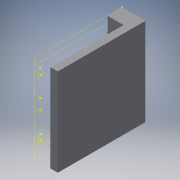
# Autodesk Inventor part: AXTS
Saved by Autodesk Inventor 2016 (Build 200138000, 138)
## iProperties
Created: 2017-07-16
Part Number: AXTS
Material: PC/ABS Plastic
Document SubType Name: Modeling
Designer: ludwi
Density: 0.357273 g/cm^3
Appearance: Smooth - White
Author: ludwi
Autodesk Inventor part; units mm, degrees
ref_plane "YZ Plane" through (0, 0, 0) normal (1, 0, 0) x (0, 1, 0)
ref_plane "XZ Plane" through (0, 0, 0) normal (0, 1, 0) x (-1, 0, 0)
ref_plane "XY Plane" through (0, 0, 0) normal (0, 0, 1) x (1, 0, 0)
sketch "Sketch1" plane through (0, 0, 0) normal (0, 0, 1) x (1, 0, 0)
  line L0 (0, 0) -> (32, 0)
  line L1 (32, 0) -> (32, -120)
  line L2 (32, -120) -> (22, -120)
  line L3 (22, -120) -> (22, -20)
  line L4 (22, -20) -> (0, -20)
  line L5 (0, -20) -> (0, 0)
  dimension "d3" = 120
  dimension "d4" = 10
  dimension "d5" = 22
  dimension "d8" = 20
  constraints: 12 end point, 4 perpendicular, 1 horizontal, 1 vertical
  measures "d3" distance of L0.end L1.end
  measures "d4" distance of L1.end L2.end
  measures "d5" horizontal distance of L0.start L2.end
  measures "d8" distance of L4.end L0.start
extrude "Extrusion1" add sketch "Sketch1" against normal blind 120
sketch "Sketch3" plane through (0, -20, 0) normal (-1, 0, 0) x (0, 0, 1)
  line L0 (-110, -97.8692) -> (-110, 18.1308) construction
  line L1 (-10, 18.1308) -> (-10, -97.8692) construction
  line L2 (-25, 8.9558) -> (-17, 8.9558) construction
  arc A0 (-17, 8.9558) -> (-17, 15.0558) centre (-17, 12.0058) ccw construction
  line L3 (-17, 15.0558) -> (-25, 15.0558) construction
  arc A1 (-25, 15.0558) -> (-25, 8.9558) centre (-25, 12.0058) ccw construction
  line L4 (-25, -94.7942) -> (-17, -94.7942) construction
  arc A2 (-17, -94.7942) -> (-17, -88.6942) centre (-17, -91.7442) ccw construction
  line L5 (-17, -88.6942) -> (-25, -88.6942) construction
  arc A3 (-25, -88.6942) -> (-25, -94.7942) centre (-25, -91.7442) ccw construction
  circle A4 centre (-25, -50.2442) radius 3.05 construction
  circle A5 centre (-25, -29.4942) radius 3.05 construction
  circle A6 centre (-95, -29.4942) radius 3.05 construction
  circle A7 centre (-95, -50.2442) radius 3.05 construction
  line L6 (-95, 15.0558) -> (-103, 15.0558) construction
  arc A8 (-103, 15.0558) -> (-103, 8.9558) centre (-103, 12.0058) ccw construction
  line L7 (-103, 8.9558) -> (-95, 8.9558) construction
  arc A9 (-95, 8.9558) -> (-95, 15.0558) centre (-95, 12.0058) ccw construction
  circle A10 centre (-67.125, 12.0058) radius 3.05 construction
  line L8 (-52.875, -32.5442) -> (-44.875, -32.5442) construction
  arc A11 (-44.875, -32.5442) -> (-44.875, -26.4442) centre (-44.875, -29.4942) ccw construction
  line L9 (-44.875, -26.4442) -> (-52.875, -26.4442) construction
  arc A12 (-52.875, -26.4442) -> (-52.875, -32.5442) centre (-52.875, -29.4942) ccw construction
  circle A13 centre (-52.875, -91.7442) radius 3.05 construction
  circle A14 centre (-52.875, 12.0058) radius 3.05 construction
  line L10 (-52.875, -53.2942) -> (-44.875, -53.2942) construction
  arc A15 (-44.875, -53.2942) -> (-44.875, -47.1942) centre (-44.875, -50.2442) ccw construction
  line L11 (-44.875, -47.1942) -> (-52.875, -47.1942) construction
  arc A16 (-52.875, -47.1942) -> (-52.875, -53.2942) centre (-52.875, -50.2442) ccw construction
  circle A17 centre (-67.125, -91.7442) radius 3.05 construction
  line L12 (-75.125, -53.2942) -> (-67.125, -53.2942) construction
  arc A18 (-67.125, -53.2942) -> (-67.125, -47.1942) centre (-67.125, -50.2442) ccw construction
  line L13 (-67.125, -47.1942) -> (-75.125, -47.1942) construction
  arc A19 (-75.125, -47.1942) -> (-75.125, -53.2942) centre (-75.125, -50.2442) ccw construction
  line L14 (-103, -94.7942) -> (-95, -94.7942) construction
  arc A20 (-95, -94.7942) -> (-95, -88.6942) centre (-95, -91.7442) ccw construction
  line L15 (-95, -88.6942) -> (-103, -88.6942) construction
  arc A21 (-103, -88.6942) -> (-103, -94.7942) centre (-103, -91.7442) ccw construction
  line L16 (-75.125, -32.5442) -> (-67.125, -32.5442) construction
  arc A22 (-67.125, -32.5442) -> (-67.125, -26.4442) centre (-67.125, -29.4942) ccw construction
  line L17 (-67.125, -26.4442) -> (-75.125, -26.4442) construction
  arc A23 (-75.125, -26.4442) -> (-75.125, -32.5442) centre (-75.125, -29.4942) ccw construction
  line L18 (0, -100) -> (0, 0) construction
  line L19 (0, 0) -> (-120, 0) construction
  line L20 (-120, -100) -> (-120, 0) construction
  line L21 (0, -100) -> (-120, -100) construction
  line L22 (0, 0) -> (0, 20) construction
  line L23 (0, 20) -> (-120, 20) construction
  line L24 (-120, 0) -> (-120, 20) construction
  line L25 (0, 0) -> (-120, 0) construction
  line L26 (-120, 0) -> (-110, -10)
  line L27 (-110, -99.8692) -> (-110, -10)
  line L28 (0, -100) -> (-120, -100) projected
  line L29 (-120, -100) -> (-110, -99.8692)
  line L30 (-120, -100) -> (-120, 0)
  line L31 (-120, 20) -> (-120, -100) projected
  line L32 (0, 0) -> (-120, 0) projected
  line L33 (0, 0) -> (-10, -10)
  line L34 (-10, -10) -> (-10, -99.8692)
  line L35 (0, 20) -> (0, -100) projected
  line L36 (-10, -99.8692) -> (0, -100)
  line L37 (0, -100) -> (0, -100)
  line L38 (0, 0) -> (0, -100)
  line L39 (-120, -98.4303) -> (-110, -98.4303)
  line L40 (-110, -98.4303) -> (-110, -107.1574)
  line L41 (-110, -107.1574) -> (-120, -107.1574)
  line L42 (-120, -107.1574) -> (-120, -98.4303)
  line L43 (0, -94.7942) -> (-10, -94.7942)
  line L44 (-10, -94.7942) -> (-10, -110)
  line L45 (-10, -110) -> (0, -110)
  line L46 (0, -110) -> (0, -94.7942)
  line L47 (-10, 18.1308) -> (-110, 18.1308) projected
  line L48 (-110, -97.8692) -> (-10, -97.8692) projected
  point P0 (-213, 15.0558)
  point P1 (-213, -88.6942)
  point P2 (-127, 8.9558)
  point P3 (-185.125, -26.4442)
  point P4 (-185.125, -47.1942)
  point P5 (-162.875, -47.1942)
  point P6 (-135, -88.6942)
  point P7 (-162.875, -26.4442)
  dimension "d12" = 135
  dimension "d13" = 135
  constraints: 34 end point, 4 parallel, 4 point on line, 3 perpendicular, 2 collinear, 2 horizontal
  measures "d12" angle of L35 L33
  measures "d13" angle of L20 L26
extrude "Extrusion2" cut sketch "Sketch3" against normal through all contours L26 L27 L39 L30 | L39 L27 L29 L30 | L35 L43 L34 L33 | L29 L40 L28 | L28 L40 L41 L42 | L35 L36 L34 L43 | L46 L45 L44 L28 | L28 L44 L36
chamfer "Chamfer2" distance 2 angle 45 6 edges at (22, -20, -60) (0, -20, -60) (0, 0, -60) (32, 0, -60) (32, -120, -60) (22, -120, -60)
sketch "Sketch4" plane through (2, -20, -120) normal (0, -1, 0) x (1, 0, 0)
  line L0 (98.1462, 2) -> (-1.8538, 2) construction
  line L1 (98.1462, 2) -> (98.1462, 118) construction
  line L2 (-1.8538, 118) -> (98.1462, 118) construction
  line L3 (-1.8538, 118) -> (-1.8538, 2) construction
  line L4 (83.1462, 11.175) -> (91.1462, 11.175) construction
  arc A0 (91.1462, 5.075) -> (91.1462, 11.175) centre (91.1462, 8.125) ccw construction
  line L5 (91.1462, 5.075) -> (83.1462, 5.075) construction
  arc A1 (83.1462, 11.175) -> (83.1462, 5.075) centre (83.1462, 8.125) ccw construction
  line L6 (83.1462, 114.925) -> (91.1462, 114.925) construction
  arc A2 (91.1462, 108.825) -> (91.1462, 114.925) centre (91.1462, 111.875) ccw construction
  line L7 (91.1462, 108.825) -> (83.1462, 108.825) construction
  arc A3 (83.1462, 114.925) -> (83.1462, 108.825) centre (83.1462, 111.875) ccw construction
  circle A4 centre (83.1462, 70.375) radius 3.05 construction
  circle A5 centre (83.1462, 49.625) radius 3.05 construction
  circle A6 centre (13.1462, 49.625) radius 3.05 construction
  circle A7 centre (13.1462, 70.375) radius 3.05 construction
  line L8 (13.1462, 5.075) -> (5.1462, 5.075) construction
  arc A8 (5.1462, 11.175) -> (5.1462, 5.075) centre (5.1462, 8.125) ccw construction
  line L9 (5.1462, 11.175) -> (13.1462, 11.175) construction
  arc A9 (13.1462, 5.075) -> (13.1462, 11.175) centre (13.1462, 8.125) ccw construction
  circle A10 centre (41.0212, 8.125) radius 3.05 construction
  line L10 (55.2712, 52.675) -> (63.2712, 52.675) construction
  arc A11 (63.2712, 46.575) -> (63.2712, 52.675) centre (63.2712, 49.625) ccw construction
  line L11 (63.2712, 46.575) -> (55.2712, 46.575) construction
  arc A12 (55.2712, 52.675) -> (55.2712, 46.575) centre (55.2712, 49.625) ccw construction
  circle A13 centre (55.2712, 111.875) radius 3.05 construction
  circle A14 centre (55.2712, 8.125) radius 3.05 construction
  line L12 (55.2712, 73.425) -> (63.2712, 73.425) construction
  arc A15 (63.2712, 67.325) -> (63.2712, 73.425) centre (63.2712, 70.375) ccw construction
  line L13 (63.2712, 67.325) -> (55.2712, 67.325) construction
  arc A16 (55.2712, 73.425) -> (55.2712, 67.325) centre (55.2712, 70.375) ccw construction
  circle A17 centre (41.0212, 111.875) radius 3.05 construction
  line L14 (33.0212, 73.425) -> (41.0212, 73.425) construction
  arc A18 (41.0212, 67.325) -> (41.0212, 73.425) centre (41.0212, 70.375) ccw construction
  line L15 (41.0212, 67.325) -> (33.0212, 67.325) construction
  arc A19 (33.0212, 73.425) -> (33.0212, 67.325) centre (33.0212, 70.375) ccw construction
  line L16 (5.1462, 114.925) -> (13.1462, 114.925) construction
  arc A20 (13.1462, 108.825) -> (13.1462, 114.925) centre (13.1462, 111.875) ccw construction
  line L17 (13.1462, 108.825) -> (5.1462, 108.825) construction
  arc A21 (5.1462, 114.925) -> (5.1462, 108.825) centre (5.1462, 111.875) ccw construction
  line L18 (33.0212, 52.675) -> (41.0212, 52.675) construction
  arc A22 (41.0212, 46.575) -> (41.0212, 52.675) centre (41.0212, 49.625) ccw construction
  line L19 (41.0212, 46.575) -> (33.0212, 46.575) construction
  arc A23 (33.0212, 52.675) -> (33.0212, 46.575) centre (33.0212, 49.625) ccw construction
  line L20 (13.1462, 49.625) -> (5.1462, 49.625) construction
  line L21 (13.1462, 46.575) -> (5.1462, 46.575)
  line L22 (5.1462, 52.675) -> (13.1462, 52.675)
  arc A24 (13.1462, 46.575) -> (13.1462, 52.675) centre (13.1462, 49.625) ccw
  arc A25 (5.1462, 52.675) -> (5.1462, 46.575) centre (5.1462, 49.625) ccw
  line L23 (13.1462, 70.375) -> (5.1462, 70.375) construction
  line L24 (13.1462, 67.325) -> (5.1462, 67.325)
  line L25 (5.1462, 73.425) -> (13.1462, 73.425)
  arc A26 (13.1462, 67.325) -> (13.1462, 73.425) centre (13.1462, 70.375) ccw
  arc A27 (5.1462, 73.425) -> (5.1462, 67.325) centre (5.1462, 70.375) ccw
  line L26 (13.1462, 111.875) -> (5.1462, 111.875) construction
  line L27 (13.1462, 108.825) -> (5.1462, 108.825)
  line L28 (5.1462, 114.925) -> (13.1462, 114.925)
  arc A28 (13.1462, 108.825) -> (13.1462, 114.925) centre (13.1462, 111.875) ccw
  arc A29 (5.1462, 114.925) -> (5.1462, 108.825) centre (5.1462, 111.875) ccw
  line L29 (13.1462, 8.125) -> (5.1462, 8.125) construction
  line L30 (13.1462, 5.075) -> (5.1462, 5.075)
  line L31 (5.1462, 11.175) -> (13.1462, 11.175)
  arc A30 (13.1462, 5.075) -> (13.1462, 11.175) centre (13.1462, 8.125) ccw
  arc A31 (5.1462, 11.175) -> (5.1462, 5.075) centre (5.1462, 8.125) ccw
  point P0 (-2, 120)
  point P1 (9.1462, 49.625)
  point P2 (9.1462, 70.375)
  point P3 (9.1462, 111.875)
  point P4 (9.1462, 8.125)
  constraints: 32 end point, 16 point on circle, 16 tangent, 8 centre point, 7 parallel, 4 midpoint, 2 concentric, 1 horizontal
sketch "Sketch5" plane through (22, -118, -10) normal (-1, 0, 0) x (0, 0, 1)
  line L0 (0, 116.1308) -> (-100, 116.1308) projected
  line L1 (0, 116.1308) -> (0, 0.1308) projected
  line L2 (-100, 0.1308) -> (0, 0.1308) projected
  line L3 (-100, 0.1308) -> (-100, 116.1308) projected
  line L4 (-15, 106.9558) -> (-7, 106.9558) projected
  arc A0 (-7, 106.9558) -> (-7, 113.0558) centre (-7, 110.0058) ccw projected
  line L5 (-7, 113.0558) -> (-15, 113.0558) projected
  arc A1 (-15, 113.0558) -> (-15, 106.9558) centre (-15, 110.0058) ccw projected
  line L6 (-15, 3.2058) -> (-7, 3.2058) projected
  arc A2 (-7, 3.2058) -> (-7, 9.3058) centre (-7, 6.2558) ccw projected
  line L7 (-7, 9.3058) -> (-15, 9.3058) projected
  arc A3 (-15, 9.3058) -> (-15, 3.2058) centre (-15, 6.2558) ccw projected
  circle A4 centre (-15, 47.7558) radius 3.05 projected
  circle A5 centre (-15, 68.5058) radius 3.05 projected
  circle A6 centre (-85, 68.5058) radius 3.05 projected
  circle A7 centre (-85, 47.7558) radius 3.05 projected
  line L8 (-85, 113.0558) -> (-93, 113.0558) projected
  arc A8 (-93, 113.0558) -> (-93, 106.9558) centre (-93, 110.0058) ccw projected
  line L9 (-93, 106.9558) -> (-85, 106.9558) projected
  arc A9 (-85, 106.9558) -> (-85, 113.0558) centre (-85, 110.0058) ccw projected
  circle A10 centre (-57.125, 110.0058) radius 3.05 projected
  line L10 (-42.875, 65.4558) -> (-34.875, 65.4558) projected
  arc A11 (-34.875, 65.4558) -> (-34.875, 71.5558) centre (-34.875, 68.5058) ccw projected
  line L11 (-34.875, 71.5558) -> (-42.875, 71.5558) projected
  arc A12 (-42.875, 71.5558) -> (-42.875, 65.4558) centre (-42.875, 68.5058) ccw projected
  circle A13 centre (-42.875, 6.2558) radius 3.05 projected
  circle A14 centre (-42.875, 110.0058) radius 3.05 projected
  line L12 (-42.875, 44.7058) -> (-34.875, 44.7058) projected
  arc A15 (-34.875, 44.7058) -> (-34.875, 50.8058) centre (-34.875, 47.7558) ccw projected
  line L13 (-34.875, 50.8058) -> (-42.875, 50.8058) projected
  arc A16 (-42.875, 50.8058) -> (-42.875, 44.7058) centre (-42.875, 47.7558) ccw projected
  circle A17 centre (-57.125, 6.2558) radius 3.05 projected
  line L14 (-65.125, 44.7058) -> (-57.125, 44.7058) projected
  arc A18 (-57.125, 44.7058) -> (-57.125, 50.8058) centre (-57.125, 47.7558) ccw projected
  line L15 (-57.125, 50.8058) -> (-65.125, 50.8058) projected
  arc A19 (-65.125, 50.8058) -> (-65.125, 44.7058) centre (-65.125, 47.7558) ccw projected
  line L16 (-93, 3.2058) -> (-85, 3.2058) projected
  arc A20 (-85, 3.2058) -> (-85, 9.3058) centre (-85, 6.2558) ccw projected
  line L17 (-85, 9.3058) -> (-93, 9.3058) projected
  arc A21 (-93, 9.3058) -> (-93, 3.2058) centre (-93, 6.2558) ccw projected
  line L18 (-65.125, 65.4558) -> (-57.125, 65.4558) projected
  arc A22 (-57.125, 65.4558) -> (-57.125, 71.5558) centre (-57.125, 68.5058) ccw projected
  line L19 (-57.125, 71.5558) -> (-65.125, 71.5558) projected
  arc A23 (-65.125, 71.5558) -> (-65.125, 65.4558) centre (-65.125, 68.5058) ccw projected
  point P0 (10, 118)
extrude "Extrusion3" cut sketch "Sketch5" against normal through all contours A3 L7 A2 L6 | A4 | A5 | A6 | A7 | A12 L11 A11 L10 | A13 | A16 L13 A15 L12 | A17 | A19 L15 A18 L14 | A21 L17 A20 L16 | A23 L19 A22 L18
extrude "Extrusion4" cut sketch "Sketch4" against normal through all
body "Solid1"
